Autodesk Fusion 360 part; units mm, degrees
note: some values were not read from the file. Chosen so that the rebuilt part matches the saved one: which face or edge a step refers to. Set by a fixed rule: which sketch regions a step uses.
(part 2 of 2)
equation "d240 = thickframe"
equation "d242 = thickdraw / 2 + 1 mm"
equation "seconddrawerheight = drawerheight * 2"
named bodies: "Frame-top", "Frame-bottom", "Frame-left", "Frame-right", "Vertical-separator", "Fixture1", "Fixture2", "Horizontal-separator1", "Fixture3", "Fixture4", "Cleat5", "Cleat6", "Cleat7", "Cleat8", "Cleat9", "Cleat10", "Cleat11", "Cleat12", "Horizontal-separator2", "Cleat1", "Cleat2", "Cleat3", "Cleat4"
